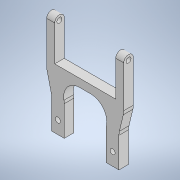
# Autodesk Inventor part: Стойка для камеры
Saved by Autodesk Inventor 2020 (Build 240168000, 168)
## iProperties
Created: 2021-04-12
Part Number: Стойка для камеры
Material: Типовые
Document SubType Name: Обычные детали
Designer: Антон
Density: 1 g/cm^3
Appearance: По умолчанию
Sheet Metal Rule: По умолчанию
Author: Антон
Autodesk Inventor part; units mm, degrees
ref_plane "YZ Plane" through (0, 0, 0) normal (1, 0, 0) x (0, 1, 0)
ref_plane "XZ Plane" through (0, 0, 0) normal (0, 1, 0) x (-1, 0, 0)
sketch "Эскиз1" plane through (0, 0, 0) normal (0, 0, 1) x (1, 0, 0)
  line L0 (0, 0) -> (5, 0)
  line L1 (5, 0) -> (5, 18)
  line L2 (5, 18) -> (0, 18)
  line L3 (0, 18) -> (0, 0)
  line L4 (0, 0) -> (24.15, 0)
  line L5 (24.15, 0) -> (24.15, -5)
  line L6 (24.15, -5) -> (0, -5)
  line L7 (0, -5) -> (0, 0)
  dimension "d0" = 5
  dimension "d1" = 18
  dimension "d2" = 24.15
  dimension "d3" = 5
  constraints: 16 end point, 4 parallel, 2 horizontal, 2 perpendicular
  measures "d0" distance of L2.end L1.end
  measures "d1" distance of L1.end L0.end
  measures "d2" distance of L5.end L6.end
  measures "d3" distance of L4.end L5.end
extrude "Выдавливание1" add sketch "Эскиз1" along normal blind 6
sketch "Эскиз4" plane through (0, 18, 0) normal (0, 1, 0) x (1, 0, 0)
  line L0 (0, 0) -> (0, -6) projected
  line L1 (0, 0) -> (0, -6) projected
  line L2 (5, 0) -> (0, 0) projected
  line L3 (0, 0) -> (0, -6) projected
  line L4 (5, -6) -> (0, -6) projected
  line L5 (5, 0) -> (5, -6) projected
extrude "Выдавливание2" add sketch "Эскиз4" along normal blind 7.2
fillet "Сопряжение1" radius 3 2 edges at (2.5, 25.2, 6) (2.5, 25.2, 0)
sketch "Эскиз5" plane through (5, 0, 6) normal (1, 0, 0) x (0, 0, -1)
  line L0 (0, -5) -> (0, -5) projected
  arc A0 (6, 22.2) -> (0, 22.2) centre (3, 22.2) ccw projected
  point P0 (6, 0)
  point P1 (6, -5)
  point P2 (2.5, 25.2)
  constraints: 2 other
hole "Отверстие2" at (5, 22.2, 3) direction (-1, 0, 0) diameter 3.2 depth 5
mirror "Зеркальное отражение1" about plane through (24.15, -5, 0) normal (1, 0, 0)
sketch "Эскиз9" plane through (0, 0, 0) normal (0, 0, -1) x (-1, 0, 0)
  line L0 (0, -5) -> (-48.3, -5) projected
  line L1 (-48.3, 22.2) -> (-48.3, -5) projected
  line L2 (-48.3, -5) -> (-45.3, -17.45)
  line L3 (-45.3, -17.45) -> (-45.3, -37.45)
  line L4 (-45.3, -37.45) -> (-37.3, -37.45)
  line L5 (-37.3, -37.45) -> (-37.3, -17.45)
  line L6 (-37.3, -17.45) -> (-40.3, -5)
  point P0 (0, 0)
  point P1 (-40.3, -5)
  dimension "d82" = 32.45
  dimension "d83" = 8
  dimension "d86" = 20
  dimension "d93" = 3
  constraints: 10 end point, 4 parallel, 2 perpendicular
  measures "d82" distance between parallel lines of L0 L4
  measures "d83" distance between parallel lines of L5 L3
  measures "d86" distance from line of L5.end L4
  measures "d93" distance between parallel lines of L1 L3
extrude "Выдавливание4" add sketch "Эскиз9" against normal blind 6
sketch "Эскиз11" plane through (0, 0, 6) normal (0, 0, 1) x (1, 0, 0)
  line L0 (41.3, -37.45) -> (41.3, -29.5)
  line L1 (37.3, -37.45) -> (45.3, -37.45) projected
  point P0 (0, 0)
  dimension "d91" = 7.95
  constraints: 2 end point, 1 midpoint, 1 perpendicular
  measures "d91" distance of L0.start L0.end
hole "Отверстие6" at (41.3, -29.5, 6) direction (0, 0, -1) diameter 3.2 end through all
ref_plane "РабПлоскость1" through (24.15, 22.2, 3) normal (1, 0, 0) x (0, 0, -1)
mirror "Зеркальное отражение2" about plane through (24.15, 22.2, 3) normal (1, 0, 0) of "Выдавливание4", "Отверстие6"
fillet "Сопряжение3" radius 10 8 edges at (45.3, -17.45, 3) (37.3, -17.45, 3) (11, -17.45, 3) (3, -17.45, 3) (0, -5, 3) (8, -5, 3) (40.3, -5, 3) (48.3, -5, 3)
equation "\"Радиус_гибки\" = Толщина"
equation "\"Ширина_просечки\" = Толщина"
equation "\"Глубина_просечки\" = 0.5 * Толщина"
equation "\"Размер_просечки\" = 4 * Толщина"
equation "\"Мин_остаток\" = 2 * Толщина"
equation "\"Радиус_перехода\" = Радиус_гибки"
equation "\"Радиус_Якоби\" = Толщина"
equation "\"Размер_зазора\" = Толщина"
equation "\"Толщина\" = 0.5"
